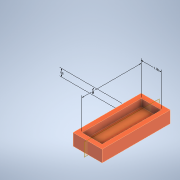
# Autodesk Inventor part: connectorToTubeBrackets
Saved by Autodesk Inventor 2021 (Build 250183000, 183)
## iProperties
Created: 2020-07-21
Part Number: connectorToTubeBrackets
Material: PC/ABS Plastic
Document SubType Name: Modeling
Designer: robst
Density: 0.357273 g/cm^3
Appearance: Smooth - Light Orange
Author: robst
Autodesk Inventor part; units mm, degrees
ref_plane "XZ Plane" through (0, 0, 0) normal (0, 1, 0) x (-1, 0, 0)
ref_plane "XY Plane" through (0, 0, 0) normal (0, 0, 1) x (1, 0, 0)
sketch "Sketch1" plane through (0, 0, 0) normal (0, 1, 0) x (-1, 0, 0)
  line L0 (31.115, 73.025) -> (-31.115, 73.025)
  line L1 (-31.115, 73.025) -> (-31.115, -73.025)
  line L2 (-31.115, -73.025) -> (31.115, -73.025)
  line L3 (31.115, -73.025) -> (31.115, 73.025)
  line L4 (31.115, 73.025) -> (-31.115, -73.025) construction
  line L5 (-31.115, 73.025) -> (31.115, -73.025) construction
  point P0 (0, 0)
  dimension "outerWidth" = 62.23
  dimension "outerLength" = 146.05
  constraints: 12 end point, 2 midpoint, 2 parallel, 1 horizontal, 1 perpendicular
  measures "outerWidth" distance of L1.end L2.end
  measures "outerLength" distance of L2.end L0.start
extrude "Extrusion1" add sketch "Sketch1" against normal blind 9.525
sketch "Sketch2" plane through (0, 0, 0) normal (0, 1, 0) x (1, 0, 0)
  line L0 (31.115, -73.025) -> (31.115, 73.025)
  line L1 (31.115, 73.025) -> (-31.115, 73.025)
  line L2 (-31.115, 73.025) -> (-31.115, -73.025)
  line L3 (-31.115, -73.025) -> (31.115, -73.025)
  line L4 (31.115, -73.025) -> (-31.115, 73.025) construction
  line L5 (31.115, 73.025) -> (-31.115, -73.025) construction
  line L6 (21.59, -63.5) -> (21.59, 63.5)
  line L7 (21.59, 63.5) -> (-21.59, 63.5)
  line L8 (-21.59, 63.5) -> (-21.59, -63.5)
  line L9 (-21.59, -63.5) -> (21.59, -63.5)
  line L10 (21.59, -63.5) -> (-21.59, 63.5) construction
  line L11 (21.59, 63.5) -> (-21.59, -63.5) construction
  line L12 (31.115, 73.025) -> (-31.115, 73.025) projected
  line L13 (-31.115, 73.025) -> (-31.115, -73.025) projected
  point P0 (0, 0)
  dimension "d1" = 9.525
  dimension "d5" = 9.525
  constraints: 24 end point, 4 midpoint, 4 parallel, 2 collinear, 2 perpendicular, 1 vertical
  measures "d1" distance between parallel lines of L7 L1
  measures "d5" distance between parallel lines of L2 L8
extrude "Extrusion2" add sketch "Sketch2" along normal blind 15.875
equation "\"outerWidth\" = innerWidth + 2 * wallThickness"
equation "\"outerLength\" = innerLength + 2 * wallThickness"
equation "\"d2\" = wallThickness"
equation "\"d1\" = wallThickness"
equation "\"d5\" = wallThickness"
equation "\"d4\" = outerHeight - wallThickness"
equation "\"innerLength\" = 127"
equation "\"width\" = 196.85"
equation "\"outerHeight\" = 25.4"
equation "\"wallThickness\" = 9.525"
equation "\"innerWidth\" = 43.18"
body "Solid1"
